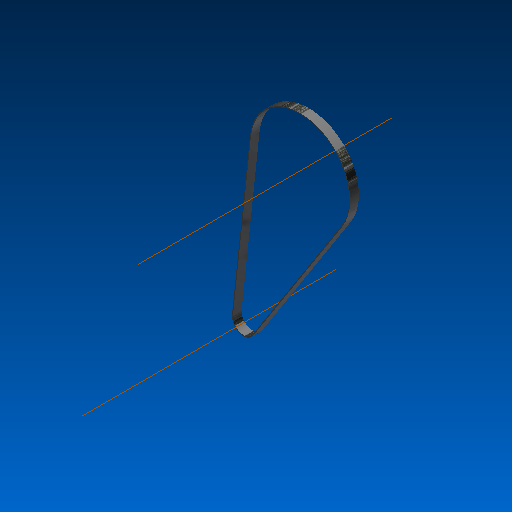
# Autodesk Inventor part: Synchronous Belt
Saved by Autodesk Inventor 2018 (Build 220112000, 112)
## iProperties
Created: 2020-07-27
Part Number: Synchronous Belt
Material: Rubber
Document SubType Name: Modeling
Designer: Bunny320
Density: 1 g/cm^3
Appearance: Rubber - Black - Version 1.1
CustomPartVersion: 1
Author: Bunny320
Autodesk Inventor part; units mm, degrees
ref_plane "YZ Plane" through (0, 0, 0) normal (1, 0, 0) x (0, 1, 0)
ref_plane "XZ Plane" through (0, 0, 0) normal (0, 1, 0) x (-1, 0, 0)
ref_plane "XY Plane" through (0, 0, 0) normal (0, 0, 1) x (1, 0, 0)
sketch "Sketch Path" plane through (0, 0, 0) normal (0, 0, 1) x (1, 0, 0)
  arc A0 (-70.1973, -62.0161) -> (-46.8226, -70.2725) centre (-57.5402, -63.399) ccw
  arc A1 (55.596, 89.4262) -> (-49.5904, 126.5803) centre (7.3664, 120.3569) ccw
  line L0 (55.596, 89.4262) -> (-46.8226, -70.2725)
  line L1 (-70.1973, -62.0161) -> (-49.5904, 126.5803)
  constraints: 4 end point, 4 point on circle, 2 centre point
ref_plane "Cross Section Plane" through (-46.8226, -70.2725, 0) normal (0.5398439, 0.8417652, 0) x (0, 0, 1)
ref_plane "Work Plane2" through (-57.5402, -63.399, 0) normal (-1, 0, 0) x (0, 0, 1)
ref_plane "Work Plane3" through (7.3664, 120.3569, 0) normal (-0.175902, -0.9844077, 0) x (0, 0, 1)
sketch "Cross Section" plane through (-46.8226, -70.2725, 0) normal (0.5398439, 0.8417652, 0) x (0, 0, 1)
  line L0 (-5, 0.5) -> (5, 0.5)
  line L1 (5, 0.5) -> (5, -0.5)
  line L2 (5, -0.5) -> (-5, -0.5)
  line L3 (-5, -0.5) -> (-5, 0.5)
  line L4 (-5, 0) -> (5, 0) construction
  point P0 (0, 0)
  point P1 (0, 0)
  dimension "d0" = 10
  dimension "d4" = 0.5
  dimension "d5" = 0.5
  constraints: 10 end point, 3 midpoint, 2 parallel, 1 coincident, 1 horizontal, 1 perpendicular, 1 other
  measures "d0" distance between parallel lines of L1 L3
  measures "d4" distance between parallel lines of L2 L4
  measures "d5" distance between parallel lines of L4 L0
sweep "Belt" add profiles "Cross Section" path "Sketch Path" path curves L1 A1 L0 A0
equation "\"d0\" = da_B"
equation "\"d4\" = da_a"
equation "\"d5\" = da_a2"
equation "\"da_B\" = 10"
equation "\"da_pb\" = 5"
equation "\"da_a\" = 0.5"
equation "\"da_S\" = 2.65"
equation "\"da_Beta\" = 20deg"
equation "\"da_Ht\" = 1.2"
equation "\"da_H\" = 2.2"
equation "\"da_a2\" = 0.5"
body "Solid1"
